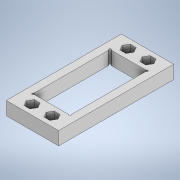
# Autodesk Inventor part: vydacha
Saved by Autodesk Inventor 2020 (Build 240168000, 168)
## iProperties
Created: 2022-07-26
Part Number: vydacha
Material: Типовые
Document SubType Name: Modeling
Designer: akapu
Density: 1 g/cm^3
Appearance: По умолчанию
Author: akapu
Autodesk Inventor part; units mm, degrees
ref_plane "YZ Plane" through (0, 0, 0) normal (1, 0, 0) x (0, 1, 0)
ref_plane "XZ Plane" through (0, 0, 0) normal (0, 1, 0) x (-1, 0, 0)
ref_plane "XY Plane" through (0, 0, 0) normal (0, 0, 1) x (1, 0, 0)
sketch "Эскиз1" plane through (0, 0, 0) normal (0, 1, 0) x (-1, 0, 0)
  line L0 (0, 0) -> (-19.5, 0)
  line L1 (-19.5, 0) -> (-19.5, -40.5)
  line L2 (-19.5, -40.5) -> (0, -40.5)
  line L3 (0, -40.5) -> (0, 0)
  line L4 (-19.5, -40.5) -> (-19.5, -45.5)
  line L5 (-19.5, -45.5) -> (-15, -45.5)
  line L6 (0, -45.5) -> (-4.5, -45.5)
  line L7 (-4.5, -45.5) -> (-15, -45.5)
  line L8 (0, -40.5) -> (-19.5, -40.5)
  line L9 (-19.5, -40.5) -> (-19.5, -50.5)
  line L10 (-19.5, -50.5) -> (0, -50.5)
  line L11 (0, -50.5) -> (0, -40.5)
  line L12 (0, 0) -> (-19.5, 0)
  line L13 (-19.5, 0) -> (-19.5, 10)
  line L14 (-19.5, 10) -> (0, 10)
  line L15 (0, 10) -> (0, 0)
  line L16 (0, 5) -> (-4.5, 5)
  line L17 (-4.5, 5) -> (-15, 5)
  line L18 (-15, 5) -> (-19.5, 5)
  line L19 (-19.5, -50.5) -> (-23.5, -50.5)
  line L20 (-23.5, -50.5) -> (-23.5, 10)
  line L21 (-23.5, 10) -> (-19.5, 10)
  line L22 (-19.5, 10) -> (-19.5, -50.5)
  line L23 (0, 10) -> (4, 10)
  line L24 (4, 10) -> (4, -50.5)
  line L25 (4, -50.5) -> (0, -50.5)
  line L26 (0, -50.5) -> (0, 10)
  circle A0 centre (-4.5, -45.5) radius 1.25
  circle A1 centre (-15, -45.5) radius 1.25
  circle A2 centre (-4.5, 5) radius 1.25
  circle A3 centre (-15, 5) radius 1.25
  circle A4 centre (0, -40.5) radius 0.5
  circle A5 centre (-19.5, -40.5) radius 0.5
  circle A6 centre (0, 0) radius 0.5
  circle A7 centre (-19.5, 0) radius 0.5
  point P0 (-19, 0)
  point P1 (-0.5, 0)
  point P2 (0, -0.5)
  point P3 (0, -40)
  point P4 (-0.5, -40.5)
  point P5 (-19, -40.5)
  point P6 (-19.5, -40)
  point P7 (-19.5, -0.5)
  dimension "d0" = 19.5
  dimension "d1" = 40.5
  dimension "d2" = 5
  dimension "d3" = 4.5
  dimension "d4" = 4.5
  dimension "d5" = 10
  dimension "d6" = 10
  dimension "d7" = 4
  dimension "d8" = 4
  dimension "d9" = 2.5
  dimension "d10" = 2.5
  dimension "d11" = 2.5
  dimension "d12" = 2.5
  dimension "d16" = 1
  dimension "d17" = 1
  dimension "d18" = 1
  dimension "d19" = 1
  constraints: 54 end point, 10 parallel, 8 centre point, 8 coincident, 7 horizontal, 6 perpendicular, 3 point on line, 2 midpoint, 1 collinear, 1 vertical
  measures "d0" distance of L2.end L1.end
  measures "d1" distance of L1.end L0.end
  measures "d2" distance of L1.end L4.end
  measures "d3" distance of L4.end L5.end
  measures "d4" distance of L6.start L6.end
  measures "d5" distance of L9.end L8.end
  measures "d6" distance of L12.end L13.end
  measures "d7" distance of L20.end L21.end
  measures "d8" distance of L24.end L25.end
  measures "d9" diameter of A0
  measures "d10" diameter of A1
  measures "d11" diameter of A2
  measures "d12" diameter of A3
  measures "d16" diameter of A4
  measures "d17" diameter of A5
  measures "d18" diameter of A6
  measures "d19" diameter of A7
extrude "Выдавливание1" add sketch "Эскиз1" along normal blind 7 contours A7 L13 L18 A3 L17 A2 L16 L15 A6 L0 | A7 L1 A5 L4 L9 L19 L20 L21 L13 | L15 L23 L24 L25 L11 A4 L3 A6 | L13 L14 L15 L16 A2 L17 A3 L18 | L2 A4 L11 L6 A0 L7 A1 L5 L4 A5 | L5 A1 L7 A0 L6 L11 L10 L9
fillet "Сопряжение1" radius 0.4 8 edges at (0, 3.5, -0.5) (0.5, 3.5, 0) (0, 3.5, -40) (0.5, 3.5, -40.5) (19.5, 3.5, -40) (19, 3.5, -40.5) (19.5, 3.5, -0.5) (19, 3.5, 0)
sketch "Эскиз2" plane through (0, 7, 0) normal (0, 1, 0) x (1, 0, 0)
  circle A0 centre (4.5, -5) radius 1.25 projected
  line L0 (4.5, -5) -> (4.5, -2.3)
  circle A1 centre (15, 45.5) radius 1.25 projected
  line L1 (15, 45.5) -> (15, 42.8)
  line L2 (13.4412, 42.8) -> (11.8823, 45.5)
  line L3 (11.8823, 45.5) -> (13.4412, 48.2)
  line L4 (13.4412, 48.2) -> (16.5588, 48.2)
  line L5 (16.5588, 48.2) -> (18.1177, 45.5)
  line L6 (18.1177, 45.5) -> (16.5588, 42.8)
  line L7 (16.5588, 42.8) -> (13.4412, 42.8)
  circle A2 centre (4.5, 45.5) radius 1.25 projected
  line L8 (2.9412, 42.8) -> (1.3823, 45.5)
  line L9 (1.3823, 45.5) -> (2.9412, 48.2)
  line L10 (2.9412, 48.2) -> (6.0588, 48.2)
  line L11 (6.0588, 48.2) -> (7.6177, 45.5)
  line L12 (7.6177, 45.5) -> (6.0588, 42.8)
  line L13 (6.0588, 42.8) -> (2.9412, 42.8)
  line L14 (6.0588, -2.3) -> (7.6177, -5)
  line L15 (7.6177, -5) -> (6.0588, -7.7)
  line L16 (6.0588, -7.7) -> (2.9412, -7.7)
  line L17 (2.9412, -7.7) -> (1.3823, -5)
  line L18 (1.3823, -5) -> (2.9412, -2.3)
  line L19 (2.9412, -2.3) -> (6.0588, -2.3)
  circle A3 centre (15, -5) radius 1.25 projected
  line L20 (16.5588, -2.3) -> (18.1177, -5)
  line L21 (18.1177, -5) -> (16.5588, -7.7)
  line L22 (16.5588, -7.7) -> (13.4412, -7.7)
  line L23 (13.4412, -7.7) -> (11.8823, -5)
  line L24 (11.8823, -5) -> (13.4412, -2.3)
  line L25 (13.4412, -2.3) -> (16.5588, -2.3)
  point P0 (0, 0)
  point P1 (4.5, 42.8)
  point P2 (15, -2.3)
  dimension "d21" = 2.7
  dimension "d22" = 2.7
  constraints: 52 end point, 4 coincident, 4 midpoint, 2 point on line, 2 vertical, 52 other
  measures "d21" distance of L0.start L0.end
  measures "d22" distance of L1.start L1.end
extrude "Выдавливание2" cut sketch "Эскиз2" against normal blind 3.5 contours A0 | L19 L14 L15 L16 L17 L18 | A1 | L7 L2 L3 L4 L5 L6 | A2 | L8 L9 L10 L11 L12 L13 | A3 | L20 L21 L22 L23 L24 L25
